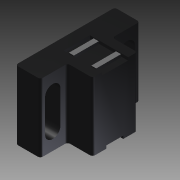
# Autodesk Inventor part: May Tec 1.65.2101_Magnetic lock PA 0
Saved by Autodesk Inventor 2016 (Build 200138000, 138)
## iProperties
Category: PARTsolutions
Company: MAYTEC
Created: 2018-04-09
Part Number: May Tec 1.65.2101_Magnetic lock PA 0
Catalog Web Link: www.cadenas.de
Description: 1.65.2101-Magnetic lock PA
Vendor: MAYTEC
Document SubType Name: Modeling
Designer: psAdmin
Manufacturer: MAYTEC
Mass: 11.2437 g
Surface Area: 54.7438 cm^2
Volume: 11.2437 cm^3
Density: 1 g/cm^3
Material: Generic
Appearance: PSOLRGB-25-25-25
PSOL_IDENT_0: {$CADENAS_DATA\23d-libs\maytec\maytec_3d\anbauzubehoer\magnetverschluss_pa\verschluss.prj},218 {VTYP=
PSOL_IDENT_1: 3D},{NB=May Tec 1.65.2101_Magnetic lock PA 0},{LINA=May Tec 1.65.2101_Magnetic lock PA 0},{NN=1.65.2
PSOL_IDENT_2: 101},{DATE=09.02.2017 10:28:49},{GEOMDATE=29.06.2009 00:00:00},{VERSION=},{LINEID=10},{LINESUBID=-1}
PSOL_IDENT_3: ,{WBVAR=L}  {NB=May Tec 1.65.2101_Magnetic lock PA 0},{LINA=May Tec 1.65.2101_Magnetic lock PA 0},{K
PSOL_IDENT_4: T=DUMMY},{PARTNR=1.65.2101},{DESCRIPTION=Magnetverschluss PA},{XTRANS=Magnetic lock PA},{L=0}
NN: 1.65.2101
NT: Magnetic lock PA
NB: May Tec 1.65.2101_Magnetic lock PA 0
NBSYN: May Tec $PARTNR._$XTRANS. $L.
LINA: May Tec 1.65.2101_Magnetic lock PA 0
PARTNR: 1.65.2101
DESCRIPTION: Magnetic lock PA
L: 0
SUPPLIER: MAYTEC
ARTICLENO: May Tec 1.65.2101_Magnetic lock PA 0
BOMINFO: May Tec 1.65.2101_Magnetic lock PA 0
CREATOR: CADENAS GmbH
Title: May Tec 1.65.2101_Magnetic lock PA 0
Author: Cadenas PARTsolutions
Comments: Magnetic lock PA
Autodesk Inventor part; units mm, degrees
sketch "Skizze_1" plane through (0, 0, 0) normal (0, 0, 1) x (1, 0, 0)
  line L0 (0, 19) -> (0, -19)
  arc A0 (0, -19) -> (1, -20) centre (1, -19) ccw
  line L1 (1, -20) -> (9, -20)
  arc A1 (9, -20) -> (10, -19) centre (9, -19) ccw
  line L2 (10, -19) -> (10, -10)
  arc A2 (11, -9) -> (10, -10) centre (11, -10) ccw
  line L3 (11, -9) -> (19, -9)
  arc A3 (19, -9) -> (20, -8) centre (19, -8) ccw
  line L4 (20, -8) -> (20, 8)
  arc A4 (20, 8) -> (19, 9) centre (19, 8) ccw
  line L5 (19, 9) -> (11, 9)
  arc A5 (10, 10) -> (11, 9) centre (11, 10) ccw
  line L6 (10, 10) -> (10, 19)
  arc A6 (10, 19) -> (9, 20) centre (9, 19) ccw
  line L7 (9, 20) -> (1, 20)
  arc A7 (1, 20) -> (0, 19) centre (1, 19) ccw
  constraints: 16 end point, 16 point on circle, 8 centre point
extrude "Extrusion1" add sketch "Skizze_1" along normal mid plane 27.5
sketch "Skizze_2" plane through (0, 0, 0) normal (1, 0, 0) x (0, 1, 0)
  arc A0 (18.1, 6.5) -> (11.9, 6.5) centre (15, 6.5) ccw
  line L0 (11.9, 6.5) -> (11.9, -6.5)
  arc A1 (11.9, -6.5) -> (18.1, -6.5) centre (15, -6.5) ccw
  line L1 (18.1, -6.5) -> (18.1, 6.5)
  constraints: 4 end point, 4 point on circle, 2 centre point
extrude "Extrusion2" cut sketch "Skizze_2" along normal blind 10
sketch "Skizze_3" plane through (0, 0, 0) normal (1, 0, 0) x (0, 1, 0)
  arc A0 (-11.9, 6.5) -> (-18.1, 6.5) centre (-15, 6.5) ccw
  line L0 (-18.1, 6.5) -> (-18.1, -6.5)
  arc A1 (-18.1, -6.5) -> (-11.9, -6.5) centre (-15, -6.5) ccw
  line L1 (-11.9, -6.5) -> (-11.9, 6.5)
  constraints: 4 end point, 4 point on circle, 2 centre point
extrude "Extrusion3" cut sketch "Skizze_3" along normal blind 10
sketch "Skizze_4" plane through (20, 0, 0) normal (1, 0, 0) x (0, 0, -1)
  line L0 (-13.75, 5.325) -> (-13.75, -5.325)
  line L1 (-13.75, -5.325) -> (-12.6, -5.325)
  line L2 (-12.6, -5.325) -> (-12.6, 5.325)
  line L3 (-12.6, 5.325) -> (-13.75, 5.325)
  constraints: 8 end point
extrude "Extrusion4" cut sketch "Skizze_4" against normal blind 15.32
sketch "Skizze_5" plane through (20, 0, 0) normal (1, 0, 0) x (0, 0, -1)
  line L0 (12.6, 3.4) -> (12.6, -3.4)
  line L1 (12.6, -3.4) -> (13.75, -3.4)
  line L2 (13.75, -3.4) -> (13.75, 3.4)
  line L3 (13.75, 3.4) -> (12.6, 3.4)
  constraints: 8 end point
extrude "Extrusion5" cut sketch "Skizze_5" against normal blind 15.32
sketch "Skizze_6" plane through (0, 0, 0) normal (0, 1, 0) x (-1, 0, 0)
  line L0 (-6.5, 8.75) -> (-6.5, 13.75)
  line L1 (-6.5, 13.75) -> (-8.5, 13.75)
  line L2 (-8.5, 13.75) -> (-8.5, 11.75)
  line L3 (-8.5, 11.75) -> (-15.5, 11.75)
  line L4 (-15.5, 11.75) -> (-15.5, 13.75)
  line L5 (-15.5, 13.75) -> (-17.5, 13.75)
  line L6 (-17.5, 13.75) -> (-17.5, 8.75)
  line L7 (-17.5, 8.75) -> (-6.5, 8.75)
  constraints: 16 end point
extrude "Extrusion6" add sketch "Skizze_6" along normal mid plane 10
sketch "Skizze_7" plane through (0, 0, 0) normal (0, 1, 0) x (-1, 0, 0)
  line L0 (-6.5, -8.75) -> (-17.5, -8.75)
  line L1 (-17.5, -8.75) -> (-17.5, -13.75)
  line L2 (-17.5, -13.75) -> (-15.5, -13.75)
  line L3 (-15.5, -13.75) -> (-15.5, -11.75)
  line L4 (-15.5, -11.75) -> (-8.5, -11.75)
  line L5 (-8.5, -11.75) -> (-8.5, -13.75)
  line L6 (-8.5, -13.75) -> (-6.5, -13.75)
  line L7 (-6.5, -13.75) -> (-6.5, -8.75)
  constraints: 16 end point
extrude "Extrusion7" add sketch "Skizze_7" along normal mid plane 6.75
sketch "Skizze_8" plane through (0, 0, 0) normal (1, 0, 0) x (0, 1, 0)
  line L0 (7.5, 12.425) -> (-7.5, 12.425)
  line L1 (-7.5, 12.425) -> (-7.5, -12.425)
  line L2 (-7.5, -12.425) -> (7.5, -12.425)
  line L3 (7.5, -12.425) -> (7.5, 12.425)
  constraints: 8 end point
extrude "Extrusion8" cut sketch "Skizze_8" along normal blind 6
ref_plane "side_1_XY" through (0, 0, 0) normal (-1, 0, 0) x (0, 0, -1)
ref_plane "side_1_YZ" through (0, 0, 0) normal (0, 0, -1) x (0, -1, 0)
ref_plane "side_1_ZX" through (0, 0, 0) normal (0, -1, 0) x (-1, 0, 0)
body "Solid1"
